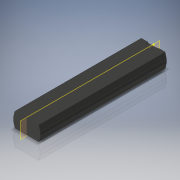
# Autodesk Inventor part: atmega_mold
Saved by Autodesk Inventor 2018 (Build 220112000, 112)
## iProperties
Created: 2017-04-13
Part Number: atmega_mold
Material: Generic
Document SubType Name: Modeling
Designer: kampe_000
Density: 1 g/cm^3
Appearance: Default
Author: kampe_000
Autodesk Inventor part; units mm, degrees
ref_plane "YZ Plane" through (0, 0, 0) normal (1, 0, 0) x (0, 1, 0)
ref_plane "XZ Plane" through (0, 0, 0) normal (0, 1, 0) x (-1, 0, 0)
ref_plane "XY Plane" through (0, 0, 0) normal (0, 0, 1) x (1, 0, 0)
sketch "Sketch1" plane through (0, 0, 0) normal (0, 1, 0) x (-1, 0, 0)
  line L0 (0, 0) -> (7.3, 0)
  line L1 (7.3, 0) -> (7.3, -34.6)
  line L2 (7.3, -34.6) -> (0, -34.6)
  line L3 (0, -34.6) -> (0, 0)
  dimension "d0" = 7.3
  dimension "d1" = 34.6
  constraints: 8 end point, 2 parallel, 1 horizontal, 1 perpendicular
  measures "d0" distance of L1.end L2.end
  measures "d1" distance of L0.end L1.end
extrude "Extrusion1" add sketch "Sketch1" along normal blind 4
chamfer "Chamfer1" distance 0.4 distance2 1.5 1 edges at (0, 4, -17.3) measured on face at (-0.5, 4, -17.3)
chamfer "Chamfer2" distance 0.4 distance2 1.5 1 edges at (0, 0, -17.3) measured on face at (-0.5, 0, -17.3)
chamfer "Chamfer3" distance 0.4 distance2 1.5 1 edges at (-7.3, 4, -17.3) measured on face at (-6.8, 4, -17.3)
chamfer "Chamfer4" distance 0.4 distance2 1.5 1 edges at (-7.3, 0, -17.3) measured on face at (-6.8, 0, -17.3)
ref_plane "Work Plane1" through (-3.65, 2.5, 0) normal (1, 0, 0) x (0, 0, -1)
hole "Hole1" at (-3.65, 4, -34.6) direction (0, -1, 0) diameter 3 depth 0.2
equation "\"d4\" = AtmegaChamfer_D1"
equation "\"d5\" = AtmegaChamfer_D2"
equation "\"d7\" = AtmegaChamfer_D1"
equation "\"d8\" = AtmegaChamfer_D2"
equation "\"d10\" = AtmegaChamfer_D1"
equation "\"d11\" = AtmegaChamfer_D2"
equation "\"d13\" = AtmegaChamfer_D1"
equation "\"d14\" = AtmegaChamfer_D2"
equation "\"AtmegaChamfer_D1\" = 0.4"
equation "\"AtmegaChamfer_D2\" = 1.5"
body "Solid1"
